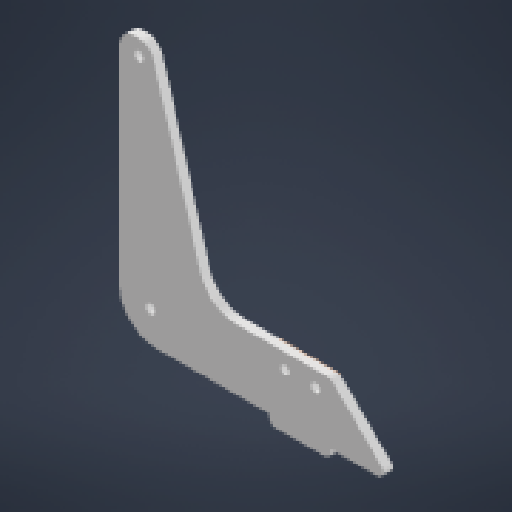
# Autodesk Inventor part: ParedLateralGrua1
Saved by Autodesk Inventor 2026.2 (Build 302298010, 298A)
## iProperties
Created: 2026-04-22
Part Number: ParedLateralGrua1
Material: Genérico
Document SubType Name: Modeling
Designer: Jose Carlos
Density: 1 g/cm^3
Appearance: Valor por defecto
Author: Jose Carlos
Autodesk Inventor part; units mm, degrees
ref_plane "YZ Plane" through (0, 0, 0) normal (1, 0, 0) x (0, 1, 0)
ref_plane "XZ Plane" through (0, 0, 0) normal (0, 1, 0) x (-1, 0, 0)
ref_plane "XY Plane" through (0, 0, 0) normal (0, 0, 1) x (1, 0, 0)
ref_plane "Plano de trabajo1" through (0, 0, 0) normal (0, 0, 1) x (1, 0, 0)
sketch "Boceto1" plane through (0, 0, 0) normal (0, 0, 1) x (1, 0, 0)
  line L0 (0, 0) -> (0, -3) construction
  line L1 (20, -3) -> (0, -3) construction
  line L2 (20, 0) -> (20, -3) construction
  line L3 (20, 0) -> (-49, 0)
  line L4 (-49, 0) -> (-49, 85) construction
  line L5 (-49, 85) -> (20, 85) construction
  line L6 (20, 85) -> (20, 0) construction
  line L7 (0, 0) -> (0, -1)
  line L8 (20, -1) -> (20, 0)
  line L9 (18, -3) -> (2, -3)
  arc A0 (0, -1) -> (2, -3) centre (2, -1) ccw
  arc A1 (18, -3) -> (20, -1) centre (18, -1) ccw
  line L10 (20, 0) -> (35.1716, 0)
  line L11 (40, 0) -> (40, 20) construction
  line L12 (40, 20) -> (20, 20) construction
  line L13 (20, 20) -> (20, 0)
  line L14 (-34, 0) -> (-34, -3) construction
  circle A2 centre (-39, 10.2728) radius 1.5
  line L15 (40, 0) -> (20, 20)
  line L16 (20, 20) -> (-49, 20)
  line L17 (-20, 20) -> (-39, 85)
  line L18 (-49, 0) -> (-49, 85)
  line L19 (-39, 85) -> (-49, 85)
  line L20 (40, 0) -> (20, 0)
  point P0 (35.1716, 0)
  dimension "d0" = 2
  dimension "d1" = 20
  dimension "d2" = 20
  dimension "d4" = 85
  dimension "d5" = 15
  dimension "d6" = 3
  dimension "d8" = 45
  dimension "d9" = 0
  dimension "d12" = 40
  dimension "d13" = 10
  constraints: 34 end point, 9 point on line, 5 parallel, 4 perpendicular, 4 point on circle, 4 tangent, 3 centre point, 3 horizontal, 1 coincident, 1 collinear, 1 equal radius, 1 vertical, 1 other
  measures "d0" radius of A0
  measures "d1" distance of L11.end L12.end
  measures "d2" distance of L11.start L11.end
  measures "d4" distance of L3.end L4.end
  measures "d5" distance between parallel lines of L14 L4
  measures "d6" diameter of A2
  measures "d8" angle of L10 L15
  measures "d9" angle of L3 L16
  measures "d12" distance from line of L6 L17.start
  measures "d13" distance of L4.end L17.end
extrude "Extrusión1" add sketch "Boceto1" along normal blind 3
fillet "Empalme1" radius 2 1 edges at (40, 0, 1.5)
fillet "Empalme2" radius 12 1 edges at (-49, 0, 1.5)
fillet "Empalme3" radius 4 1 edges at (20, 20, 1.5)
fillet "Empalme4" radius 12 1 edges at (-20, 20, 1.5)
fillet "Empalme5" radius 5 2 edges at (-39, 85, 1.5) (-49, 85, 1.5)
sketch "Boceto2" plane through (0, 0, 3) normal (0, 0, 1) x (1, 0, 0)
  circle A0 centre (15, 15) radius 1.6 construction
  circle A1 centre (5, 15) radius 1.6 construction
  arc A2 (-44, 85) -> (-49, 80) centre (-44, 80) ccw construction
  arc A3 (-37.9485, 81.4028) -> (-42.7477, 85) centre (-42.7477, 80) ccw construction
  point P0 (0, 0)
  constraints: 1 coincident
hole "Agujero1" at (5, 15, 3) at (15, 15, 3) at (-42.7477, 80, 3) direction (0, 0, -1) diameter 3 end through all
